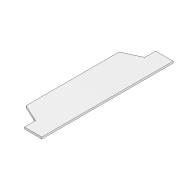
# Autodesk Inventor part: 2020-04-02-10-10201-Outline_UpperPCB
Saved by Autodesk Inventor 2020 (Build 240168000, 168)
## iProperties
Created: 2020-11-03
Part Number: 2020-04-02-10-10201-Outline_UpperPCB
Material: ABS Plastic
Document SubType Name: Modeling
Designer: eunde
Density: 1.06 g/cm^3
Appearance: Smooth - White
Author: eunde
Autodesk Inventor part; units mm, degrees
ref_plane "YZ Plane" through (0, 0, 0) normal (1, 0, 0) x (0, 1, 0)
ref_plane "XZ Plane" through (0, 0, 0) normal (0, 1, 0) x (-1, 0, 0)
ref_plane "XY Plane" through (0, 0, 0) normal (0, 0, 1) x (1, 0, 0)
sketch "Sketch1" plane through (0, 0, 0) normal (0, 1, 0) x (-1, 0, 0)
  line L0 (0, -60) -> (16, -60)
  line L1 (16, -60) -> (16, -50)
  line L2 (16, -50) -> (32, -42.5391)
  line L3 (0, -60) -> (0, 60)
  line L4 (0, 60) -> (15.7707, 60)
  line L5 (15.7707, 60) -> (15.7707, 50)
  line L6 (15.7707, 50) -> (32, 42.4322)
  line L7 (32, -42.5391) -> (32, 42.4322)
  point P0 (0, 0)
  point P1 (-7.9734, 0)
  dimension "d0" = 115
  dimension "d1" = 120
  dimension "d2" = 10
  dimension "d3" = 10
  dimension "d4" = 16
  dimension "d5" = 115
  dimension "d6" = 60
  dimension "d7" = 16
  constraints: 16 end point, 2 horizontal, 2 perpendicular, 2 vertical, 1 vertical alignment
  measures "d0" angle of L1 L2
  measures "d1" distance of L0.start L3.end
  measures "d2" distance of L0.end L1.end
  measures "d3" distance of L4.end L5.end
  measures "d4" distance of L0.start L0.end
  measures "d5" angle of L5 L6
  measures "d6" distance from line of point (-7.973, 0) L0
  measures "d7" horizontal distance of L1.end L2.end
extrude "Extrusion1" add sketch "Sketch1" along normal blind 1.6
equation "\"d3\" = d2"
equation "\"d5\" = d0"
equation "\"d6\" = 0.5 * d1"
body "Solid1"
